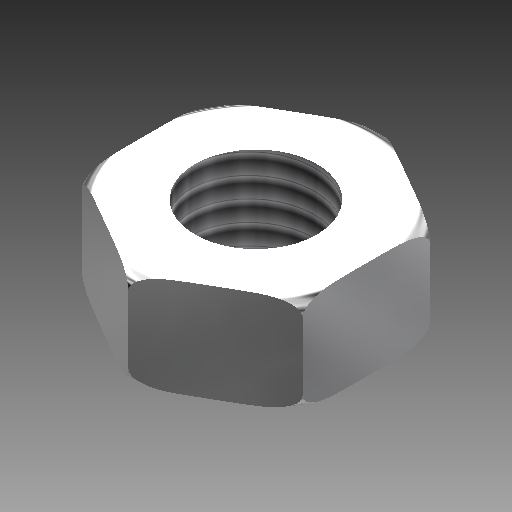
# Autodesk Inventor part: M3 nut
Saved by Autodesk Inventor 2018 (Build 220112000, 112)
## iProperties
Created: 2013-12-14
Part Number: M3 nut
Material: Generic
Document SubType Name: Modeling
Designer: beneubauer
Density: 1 g/cm^3
Appearance: Default
Author: beneubauer
Autodesk Inventor part; units mm, degrees
ref_plane "YZ Plane" through (0, 0, 0) normal (1, 0, 0) x (0, 1, 0)
ref_plane "XZ Plane" through (0, 0, 0) normal (0, 1, 0) x (-1, 0, 0)
sketch "Sketch1" plane through (0, 0, 0) normal (0, 1, 0) x (-1, 0, 0)
  line L0 (-2.7178, 1.5691) -> (0, 3.1382)
  line L1 (0, 3.1382) -> (2.7178, 1.5691)
  line L2 (2.7178, 1.5691) -> (2.7178, -1.5691)
  line L3 (2.7178, -1.5691) -> (0, -3.1382)
  line L4 (0, -3.1382) -> (-2.7178, -1.5691)
  line L5 (-2.7178, -1.5691) -> (-2.7178, 1.5691)
  circle A0 centre (0, 0) radius 1.5
  dimension "d1" = 3
  constraints: 12 end point, 2 coincident, 1 centre point, 13 other
  measures "d1" diameter of A0
extrude "Extrusion1" add sketch "Sketch1" along normal blind 2.413
thread "Thread1" size "M3x0.5" class "6H" standard "ANSI Metric M Profile" full length
sketch "Sketch3" plane through (0, 0, 0) normal (1, 0, 0) x (0, 1, 0)
  line L0 (0, 3.1382) -> (2.413, 3.1382) projected
  line L1 (0, 1.5691) -> (0, 3.1382) projected
  line L2 (0, 1.5691) -> (0, 2.7572)
  line L3 (0.381, 3.1382) -> (2.413, 3.1382)
  arc A0 (0.381, 3.1382) -> (0, 2.7572) centre (0.381, 2.7572) ccw
  line L4 (0, 2.7572) -> (-0.2163, 2.7572)
  line L5 (-0.2163, 2.7572) -> (-0.2163, 4.3172)
  line L6 (-0.2163, 4.3172) -> (0.381, 4.3172)
  line L7 (0.381, 4.3172) -> (0.381, 3.1382)
  line L8 (-0.7421, 0) -> (2.9389, 0) projected
  point P0 (0, 0)
  dimension "d8" = 0.381
  constraints: 12 end point, 3 parallel, 2 collinear, 2 point on circle, 2 point on line, 2 tangent, 1 centre point, 1 perpendicular
  measures "d8" radius of A0
ref_plane "Work Plane1" through (0, 1.2065, 3.1382) normal (0, 1, 0) x (0.866, 0, -0.5)
revolve "Revolution2" cut sketch "Sketch3" angle 360 about axis through (0, -10, 0) along (0, 1, 0)
mirror "Mirror1" about plane through (0, 1.2065, 3.1382) normal (0, 1, 0) of "Revolution2"
body "Solid1"
